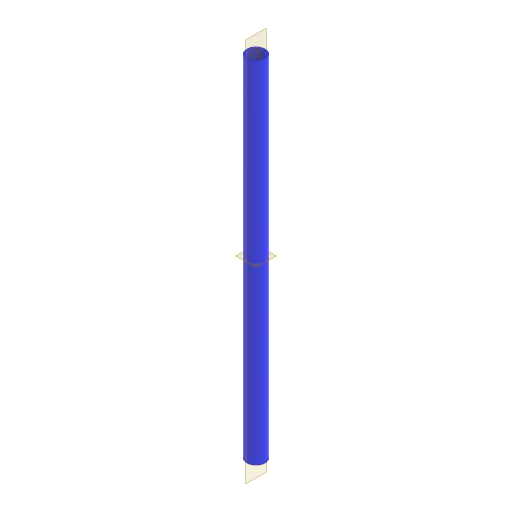
# Autodesk Inventor part: Трубка основания
Saved by Autodesk Inventor 2023.2 (Build 272271030, 271C)
## iProperties
Created: 2025-03-25
Part Number: Трубка основания
Material: Типовые
Document SubType Name: Modeling
Designer: Коноваленко
Density: 1 g/cm^3
Appearance: По умолчанию
Author: Коноваленко
Autodesk Inventor part; units mm, degrees
ref_plane "XY Plane" through (0, 0, 0) normal (0, 0, 1) x (1, 0, 0)
sketch "Эскиз1" plane through (0, 0, 0) normal (0, 1, 0) x (-1, 0, 0)
  circle A0 centre (0, 0) radius 5
  circle A1 centre (0, 0) radius 4
  dimension "d0" = 10
  dimension "d7" = 8
  constraints: 2 centre point, 2 coincident
  measures "d0" diameter of A0
  measures "d7" diameter of A1
extrude "Выдавливание1" add sketch "Эскиз1" along normal mid plane 189
sketch "Эскиз4" plane through (0, 0, 0) normal (1, 0, 0) x (0, 1, 0)
  line L0 (-94.5, 5) -> (94.5, 5) projected
  line L1 (-7.6165, -5) -> (7.6165, -5)
  line L2 (7.6165, -5) -> (7.6165, 5)
  line L3 (7.6165, 5) -> (-7.6165, 5)
  line L4 (-7.6165, 5) -> (-7.6165, -5)
  line L5 (-7.6165, -5) -> (7.6165, 5) construction
  line L6 (7.6165, -5) -> (-7.6165, 5) construction
  line L7 (0, 7) -> (0, -7) projected
  point P0 (0, 0)
  point P1 (0, 0)
  point P2 (0, 0)
  point P3 (-7.6165, 5)
  dimension "d11" = 15.233
  dimension "d12" = 10
  constraints: 12 end point, 3 midpoint, 2 parallel, 1 horizontal, 1 perpendicular, 1 point on line
  measures "d11" distance of L3.end L2.end
  measures "d12" distance of L1.end L2.end
extrude "Выдавливание3" [suppressed]
fillet "Сопряжение1" [suppressed]
